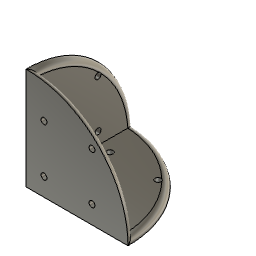
_acrylic bracket inside.18a708f7-b253-4928-abd1-c462924826e3 (Autodesk Fusion 360 design; units mm, degrees)
Autodesk Fusion 360 part; units mm, degrees
sketch "Sketch1" plane through (0, 0, 0) normal (0, 0, 1) x (1, 0, 0)
  circle A0 centre (0, 0) radius 85
  line L0 (0, 0) -> (85, 0)
  line L1 (85, 0) -> (85, 85)
  line L2 (85, 85) -> (0, 85)
  line L3 (0, 85) -> (0, 0)
  dimension "d1" = 170
  dimension "d2" = 85
  dimension "d3" = 85
  constraint coincident A0.centre L0.start
  constraint horizontal L0
  constraint vertical L1
  constraint horizontal L2
  constraint vertical L3
  measures "d1" diameter of A0
  measures "d2" distance of A0.centre L0.end
  measures "d3" distance of A0.centre L2.end
extrude "Extrude1" add sketch "Sketch1" along normal blind 5 contours A0 L0 L3 picked at (4.0323, 56.3783)
sketch "Sketch3" plane through (0, 0, 0) normal (1, 0, 0) x (0, 1, 0)
  circle A0 centre (0, 0) radius 85
  line L0 (0, 0) -> (85, 0)
  line L1 (85, 0) -> (85, 85)
  line L2 (85, 85) -> (0, 85)
  line L3 (0, 85) -> (0, 0)
  dimension "d6" = 170
  dimension "d7" = 85
  dimension "d8" = 85
  constraint coincident A0.centre L0.start
  constraint horizontal L0
  constraint vertical L1
  constraint horizontal L2
  constraint vertical L3
  measures "d6" diameter of A0
  measures "d7" distance of A0.centre L0.end
  measures "d8" distance of A0.centre L2.end
extrude "Extrude2" add sketch "Sketch3" along normal blind 5 contours A0 L0 L3 picked at (4.0323, 56.3783)
sketch "Sketch4" plane through (0, 0, 0) normal (0, 1, 0) x (1, 0, 0)
  circle A0 centre (0, 0) radius 85
  line L0 (0, 0) -> (85, 0)
  line L1 (85, 0) -> (85, -85)
  line L2 (85, -85) -> (0, -85)
  line L3 (0, -85) -> (0, 0)
  dimension "d11" = 170
  dimension "d12" = 85
  dimension "d13" = 85
  constraint coincident A0.centre L0.start
  constraint horizontal L0
  constraint vertical L1
  constraint horizontal L2
  constraint vertical L3
  measures "d11" diameter of A0
  measures "d12" distance of A0.centre L0.end
  measures "d13" distance of A0.centre L2.end
extrude "Extrude3" add sketch "Sketch4" along normal blind 5 contours A0 L0 L3 picked at (56.3783, -4.0323)
sketch "Sketch5" plane through (5, 0, 0) normal (1, 0, 0) x (0, 1, 0)
  arc A0 (84.8528, 5) -> (5, 84.8528) centre (0, 0) ccw
  line L0 (5, 5) -> (15, 5)
  line L1 (15, 5) -> (15, 15)
  line L2 (15, 15) -> (5, 15)
  line L3 (5, 15) -> (5, 5)
  line L4 (15, 15) -> (55, 15)
  line L5 (55, 15) -> (55, 55)
  line L6 (55, 55) -> (15, 55)
  line L7 (15, 55) -> (15, 15)
  line L8 (5, 84.8528) -> (5, 5)
  line L9 (5, 5) -> (84.8528, 5)
  circle A1 centre (15, 55) radius 2.5
  circle A2 centre (55, 55) radius 2.5
  circle A3 centre (55, 15) radius 2.5
  circle A4 centre (15, 15) radius 2.5
  dimension "d16" = 10
  dimension "d17" = 10
  dimension "d18" = 40
  dimension "d19" = 40
  dimension "d20" = 5
  dimension "d21" = 5
  dimension "d22" = 5
  dimension "d23" = 5
  constraint horizontal L0
  constraint vertical L1
  constraint horizontal L2
  constraint vertical L3
  constraint horizontal L4
  constraint vertical L5
  constraint horizontal L6
  constraint vertical L7
  constraint coincident L6.end L7.start
  constraint coincident L5.end L6.start
  constraint coincident L4.end L5.start
  constraint coincident L1.end L2.start
  measures "d16" distance of L0.start L0.end
  measures "d17" distance of L0.start L2.end
  measures "d18" distance of L1.end L4.end
  measures "d19" distance of L1.end L6.end
  measures "d20" diameter of A1
  measures "d21" diameter of A2
  measures "d22" diameter of A3
  measures "d23" diameter of A4
extrude "Extrude4" cut sketch "Sketch5" against normal blind 5 contours L1 L2 A4 | L1 L4 A4 | L2 L7 A4 | L4 L7 A4 | L4 L5 A3 | L4 L5 A3 | L6 L7 A1 | L6 L7 A1 | L5 L6 A2 | L5 L6 A2
sketch "Sketch6" plane through (0, 5, 0) normal (0, 1, 0) x (-1, 0, 0)
  line L0 (-5, 5) -> (-5, 84.8528)
  arc A0 (-5, 84.8528) -> (-84.8528, 5) centre (0, 0) ccw
  line L1 (-84.8528, 5) -> (-5, 5)
  line L2 (-5, 5) -> (-15, 5)
  line L3 (-15, 5) -> (-15, 15)
  line L4 (-15, 15) -> (-5, 15)
  line L5 (-5, 15) -> (-5, 5)
  line L6 (-15, 15) -> (-55, 15)
  line L7 (-55, 15) -> (-55, 55)
  line L8 (-55, 55) -> (-15, 55)
  line L9 (-15, 55) -> (-15, 15)
  circle A1 centre (-55, 55) radius 2.5
  circle A2 centre (-15, 55) radius 2.5
  circle A3 centre (-55, 15) radius 2.5
  circle A4 centre (-15, 15) radius 2.5
  dimension "d26" = 10
  dimension "d27" = 10
  dimension "d28" = 40
  dimension "d29" = 40
  dimension "d30" = 5
  dimension "d31" = 5
  dimension "d32" = 5
  dimension "d33" = 5
  constraint horizontal L2
  constraint vertical L3
  constraint horizontal L4
  constraint vertical L5
  constraint coincident L0.start L1.end
  constraint horizontal L6
  constraint vertical L7
  constraint horizontal L8
  constraint vertical L9
  constraint coincident L7.end L8.start
  constraint coincident L8.end L9.start
  constraint coincident L6.end L7.start
  constraint coincident L3.end L4.start
  measures "d26" distance of L0.start L2.end
  measures "d27" distance of L0.start L4.end
  measures "d28" distance of L3.end L6.end
  measures "d29" distance of L3.end L8.end
  measures "d30" diameter of A1
  measures "d31" diameter of A2
  measures "d32" diameter of A3
  measures "d33" diameter of A4
extrude "Extrude5" cut sketch "Sketch6" against normal blind 5 contours L3 L4 A4 | L4 L9 A4 | L3 L6 A4 | L6 L9 A4 | L8 L9 A2 | L8 L9 A2 | L6 L7 A3 | L6 L7 A3 | L7 L8 A1 | L7 L8 A1
sketch "Sketch7" plane through (0, 0, 5) normal (0, 0, 1) x (-1, 0, 0)
  line L0 (-5, -5) -> (-84.8528, -5)
  arc A0 (-84.8528, -5) -> (-5, -84.8528) centre (0, 0) ccw
  line L1 (-5, -84.8528) -> (-5, -5)
  line L2 (-5, -5) -> (-15, -5)
  line L3 (-15, -5) -> (-15, -15)
  line L4 (-15, -15) -> (-5, -15)
  line L5 (-5, -15) -> (-5, -5)
  line L6 (-15, -15) -> (-55, -15)
  line L7 (-55, -15) -> (-55, -55)
  line L8 (-55, -55) -> (-15, -55)
  line L9 (-15, -55) -> (-15, -15)
  circle A1 centre (-55, -15) radius 2.5
  circle A2 centre (-15, -15) radius 2.5
  circle A3 centre (-15, -55) radius 2.5
  circle A4 centre (-55, -55) radius 2.5
  dimension "d36" = 10
  dimension "d37" = 10
  dimension "d38" = 40
  dimension "d39" = 40
  dimension "d40" = 5
  dimension "d41" = 5
  dimension "d42" = 5
  dimension "d43" = 5
  constraint horizontal L2
  constraint vertical L3
  constraint horizontal L4
  constraint vertical L5
  constraint coincident L0.start L1.end
  constraint horizontal L6
  constraint vertical L7
  constraint horizontal L8
  constraint vertical L9
  constraint coincident L6.end L7.start
  constraint coincident L3.end L4.start
  constraint coincident L9 L8.end
  constraint coincident L7.end L8.start
  constraint coincident L8.end L9.start
  measures "d36" distance of L0.start L2.end
  measures "d37" distance of L0.start L4.end
  measures "d38" distance of L3.end L6.end
  measures "d39" distance of L3.end L8.end
  measures "d40" diameter of A1
  measures "d41" diameter of A2
  measures "d42" diameter of A3
  measures "d43" diameter of A4
extrude "Extrude6" cut sketch "Sketch7" against normal blind 5 contours L3 L4 A2 | L3 L6 A2 | L4 L9 A2 | L6 L9 A2 | L6 L7 A1 | L6 L7 A1 | L8 L9 A3 | L8 L9 A3 | L7 L8 A4 | L7 L8 A4
sketch "Sketch8" plane through (0, 0, 0) normal (0, 1, 0) x (1, 0, 0)
  circle A0 centre (0, 0) radius 85
  line L0 (0, 0) -> (104.7783, 0)
  line L1 (104.7783, 0) -> (104.7783, -102.1211)
  line L2 (104.7783, -102.1211) -> (0, -102.1211)
  line L3 (0, -102.1211) -> (0, 0)
  dimension "d46" = 170
  constraint coincident A0.centre L0.start
  constraint horizontal L0
  constraint vertical L1
  constraint horizontal L2
  constraint vertical L3
  measures "d46" diameter of A0
extrude "Extrude7" cut sketch "Sketch8" along normal blind 5 contours A0 L0 L1 L2 L3
sketch "Sketch9" plane through (5, 0, 0) normal (1, 0, 0) x (0, 1, 0)
  circle A0 centre (55, 15) radius 2.5
  circle A1 centre (55, 55) radius 2.5
  circle A2 centre (15, 15) radius 2.5
  circle A3 centre (15, 55) radius 2.5
  line L0 (5, 84.8528) -> (5, 5)
  line L1 (5, 5) -> (84.8528, 5)
  arc A4 (84.8528, 5) -> (5, 84.8528) centre (0, 0) ccw
  circle A5 centre (0, 0) radius 85
  line L2 (0, 0) -> (96.1621, 0)
  line L3 (96.1621, 0) -> (96.1621, 92.8406)
  line L4 (96.1621, 92.8406) -> (0, 92.8406)
  line L5 (0, 92.8406) -> (0, 0)
  dimension "d49" = 170
  constraint concentric A4 A5
  constraint horizontal L2
  constraint vertical L3
  constraint horizontal L4
  constraint vertical L5
  constraint coincident A4.centre A5.centre
  measures "d49" diameter of A5
extrude "Extrude8" cut sketch "Sketch9" against normal blind 10 contours A4 A5 L2 L3 L4 L5
sketch "Sketch10" plane through (0, 0, 0) normal (0, 0, 1) x (1, 0, 0)
  circle A0 centre (0, 0) radius 85
  line L0 (0, 0) -> (97.2666, 0)
  line L1 (97.2666, 0) -> (97.2666, 99.6596)
  line L2 (97.2666, 99.6596) -> (0, 99.6596)
  line L3 (0, 99.6596) -> (0, 0)
  dimension "d52" = 170
  constraint coincident A0.centre L0.start
  constraint horizontal L0
  constraint vertical L1
  constraint horizontal L2
  constraint vertical L3
  measures "d52" diameter of A0
extrude "Extrude9" cut sketch "Sketch10" along normal blind 5 contours A0 L0 L1 L2 L3
fillet "Fillet1" radius 5 3 edges at (60.1041, 60.1041, 5) (60.1041, 5, 60.1041) (5, 60.1041, 60.1041)
